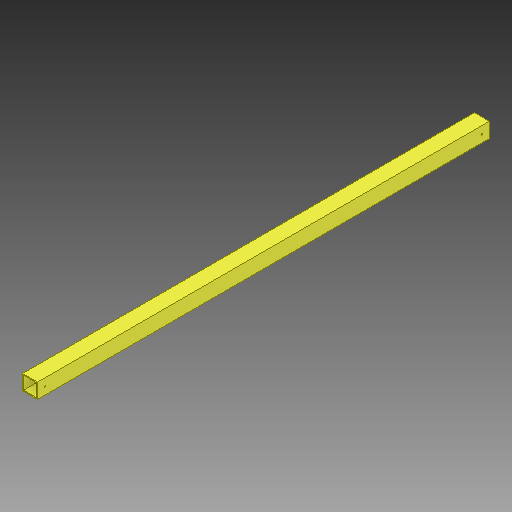
# Autodesk Inventor part: Long Side
Saved by Autodesk Inventor 2017 (Build 210142000, 142)
## iProperties
Created: 2017-01-16
Part Number: Long Side
Material: Aluminum 6061
Document SubType Name: Modeling
Designer: Ben
Density: 2.7 g/cm^3
Appearance: Smooth - Yellow
Mass: 305.739 g
Surface Area: 1430.64 cm^2
Volume: 113.237 cm^3
Author: Ben
Autodesk Inventor part; units mm, degrees
ref_plane "YZ Plane" through (0, 0, 0) normal (1, 0, 0) x (0, 1, 0)
ref_plane "XZ Plane" through (0, 0, 0) normal (0, 1, 0) x (-1, 0, 0)
ref_plane "XY Plane" through (0, 0, 0) normal (0, 0, 1) x (1, 0, 0)
sketch "Sketch1" plane through (0, 0, 0) normal (0, 0, 1) x (1, 0, 0)
  line L0 (0, 0) -> (-11.1125, 0) construction
  line L1 (0, 0) -> (0, 11.1125) construction
  line L2 (-11.1125, 11.1125) -> (11.1125, 11.1125)
  line L3 (11.1125, 11.1125) -> (11.1125, -11.1125)
  line L4 (11.1125, -11.1125) -> (-11.1125, -11.1125)
  line L5 (-11.1125, -11.1125) -> (-11.1125, 11.1125)
  line L6 (-12.7, 12.7) -> (12.7, 12.7)
  line L7 (12.7, 12.7) -> (12.7, -12.7)
  line L8 (12.7, -12.7) -> (-12.7, -12.7)
  line L9 (-12.7, -12.7) -> (-12.7, 12.7)
  line L10 (-11.1125, 0) -> (-12.7, 0) construction
  line L11 (0, 11.1125) -> (0, 12.7) construction
  dimension "d0" = 25.4
  dimension "d1" = 1.5875
  constraints: 24 end point, 4 horizontal, 4 midpoint, 4 parallel, 4 perpendicular, 2 vertical
  measures "d0" distance of L8.end L6.start
  measures "d1" distance of L1.end L11.end
extrude "Extrusion1" add sketch "Sketch1" along normal mid plane 768.35
sketch "Sketch2" plane through (12.7, -12.7, 384.175) normal (1, 0, 0) x (0, 0, -1)
  line L0 (384.175, 12.7) -> (384.175, 0) construction
  line L1 (0, 0) -> (768.35, 0) construction
  line L2 (9.525, 12.7) -> (384.175, 12.7) construction
  circle A0 centre (12.7, 12.7) radius 1.27
  circle A1 centre (755.65, 12.7) radius 1.27
  dimension "d4" = 2.54
  dimension "d6" = 12.7
  constraints: 4 end point, 2 centre point, 1 midpoint, 1 perpendicular, 1 point on line, 1 symmetric about line, 1 other
  measures "d4" diameter of A0
  measures "d6" horizontal distance of L1.start A0.centre
extrude "Extrusion2" cut sketch "Sketch2" against normal through all
body "Solid1"
